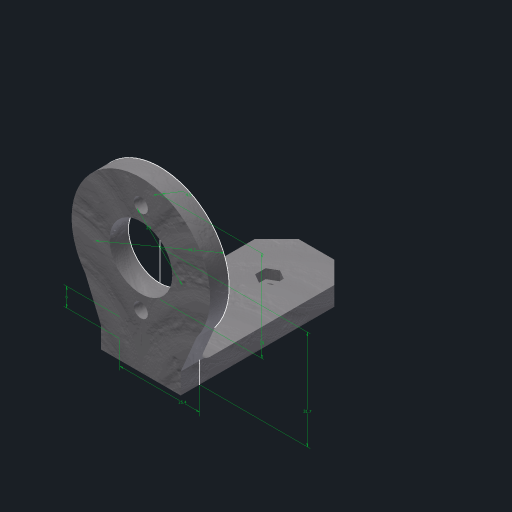
# Autodesk Inventor part: MOTOR_NUEVO_DC
Saved by Autodesk Inventor 2024.3 (Build 283343000, 343)
## iProperties
Created: 2024-08-10
Part Number: MOTOR_NUEVO_DC
Material: Steel, Mild, Welded
Document SubType Name: Modeling
Designer: Niler
Density: 7.85 g/cm^3
Appearance: Weld - Steel Mild
Author: Niler
Autodesk Inventor part; units mm, degrees
ref_plane "YZ Plane" through (0, 0, 0) normal (1, 0, 0) x (0, 1, 0)
ref_plane "XZ Plane" through (0, 0, 0) normal (0, 1, 0) x (-1, 0, 0)
ref_plane "XY Plane" through (0, 0, 0) normal (0, 0, 1) x (1, 0, 0)
sketch "Sketch1" plane through (0, 0, 0) normal (0, 0, 1) x (1, 0, 0)
  circle A0 centre (0, 0) radius 22.1
  circle A1 centre (0, 14.5) radius 2.25
  circle A2 centre (0, -14.5) radius 2.25
  line L0 (0, 14.5) -> (0, -14.5)
  circle A3 centre (0, 0) radius 10
  line L1 (-12.7, -18.0865) -> (-12.7, -31.7)
  line L2 (-12.7, -31.7) -> (12.7, -31.7)
  line L3 (12.7, -31.7) -> (12.7, -18.0865)
  line L4 (-12.7, -25.7) -> (12.7, -25.7)
  point P0 (0, -31.7)
  dimension "d0" = 44.2
  dimension "d1" = 29
  dimension "d2" = 4.5
  dimension "d3" = 20
  dimension "d4" = 31.7
  dimension "d5" = 6
  dimension "d23" = 25.4
  constraints: 10 end point, 4 centre point, 3 coincident, 3 perpendicular, 2 midpoint, 2 point on circle, 2 point on line, 2 vertical, 1 equal radius, 1 vertical alignment
  measures "d0" diameter of A0
  measures "d1" distance of L0.end L0.start
  measures "d2" diameter of A1
  measures "d3" diameter of A3
  measures "d4" distance from line of L2 point (0, 0)
  measures "d5" distance between parallel lines of L2 L4
  measures "d23" distance of L1.end L2.end
extrude "Extrusion1" add sketch "Sketch1" along normal blind 6
extrude "Extrusion2" add sketch "Sketch1" against normal blind 50 contours L4 L3 L2 L1
fillet "Fillet1" radius 3.5 1 edges at (0, -25.7, 0)
sketch "Sketch2" plane through (-12.7, -31.7, 6) normal (0, -1, 0) x (1, 0, 0)
  circle A0 centre (12.7, -41) radius 1.5
  circle A1 centre (12.7, -21) radius 1.5
  line L0 (25.4, -56) -> (0, -56) projected
  point P0 (12.7, -6)
  point P1 (12.7, -56)
  dimension "d11" = 20
  dimension "d12" = 15
  dimension "d13" = 3
  constraints: 2 centre point, 2 vertical alignment, 1 equal radius, 1 midpoint
  measures "d11" distance of A0.centre A1.centre
  measures "d12" distance from line of L0 A0.centre
  measures "d13" diameter of A0
extrude "Extrusion3" cut sketch "Sketch2" against normal blind 50
sketch "Sketch3" plane through (-12.7, -25.7, -50) normal (0, 1, 0) x (1, 0, 0)
  circle A0 centre (12.7, -35) radius 1.5 projected
  circle A1 centre (12.7, -15) radius 1.5 projected
  line L0 (25.4, -46.5) -> (0, -46.5) projected
  line L1 (25.4, -46.5) -> (25.4, 0) projected
  line L2 (0, 0) -> (25.4, 0) projected
  line L3 (0, -46.5) -> (0, 0) projected
  line L4 (12.7, -18.3486) -> (9.8, -16.6743)
  line L5 (9.8, -16.6743) -> (9.8, -13.3257)
  line L6 (9.8, -13.3257) -> (12.7, -11.6514)
  line L7 (12.7, -11.6514) -> (15.6, -13.3257)
  line L8 (15.6, -13.3257) -> (15.6, -16.6743)
  line L9 (15.6, -16.6743) -> (12.7, -18.3486)
  line L10 (12.7, -31.6514) -> (15.6, -33.3257)
  line L11 (15.6, -33.3257) -> (15.6, -36.6743)
  line L12 (15.6, -36.6743) -> (12.7, -38.3486)
  line L13 (12.7, -38.3486) -> (9.8, -36.6743)
  line L14 (9.8, -36.6743) -> (9.8, -33.3257)
  line L15 (9.8, -33.3257) -> (12.7, -31.6514)
  point P0 (12.7, -50)
  point P1 (12.7, -15)
  point P2 (12.7, -35)
  point P3 (15.6, -15)
  dimension "d16" = 5.8
  dimension "d17" = 5.8
  constraints: 24 end point, 2 coincident, 2 vertical alignment, 1 midpoint, 26 other
  measures "d16" distance from line of L5 point (15.6, -15)
  measures "d17" distance between parallel lines of L14 L11
extrude "Extrusion4" cut sketch "Sketch3" against normal blind 3 contours L4 L5 L6 L7 L8 L9 | L10 L11 L12 L13 L14 L15
chamfer "Chamfer1" distance 7 angle 45 2 edges at (12.7, -28.7, -50) (-12.7, -28.7, -50)
chamfer "Chamfer2" distance 7 angle 45 2 edges at (12.7, -18.0865, 3) (-12.7, -18.0865, 3)
body "Solid1"
